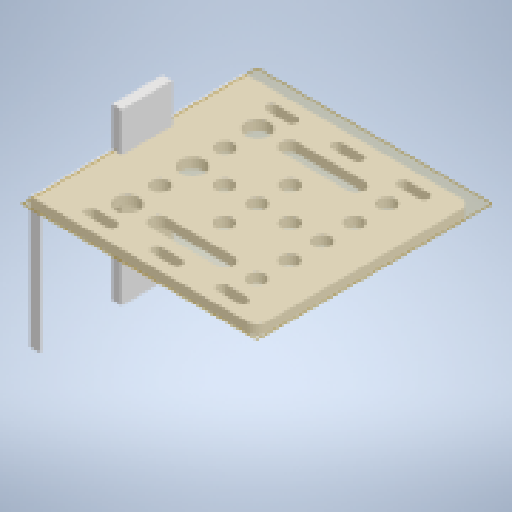
# Autodesk Inventor part: деталь основа каретки
Saved by Autodesk Inventor 2024.2 (Build 282272000, 272)
## iProperties
Created: 2026-01-31
Part Number: деталь основа каретки
Material: Типовые
Document SubType Name: Modeling
Designer: katya_notebook
Density: 1 g/cm^3
Appearance: По умолчанию
Author: katya_notebook
Autodesk Inventor part; units mm, degrees
ref_plane "YZ Plane" through (0, 0, 0) normal (1, 0, 0) x (0, 1, 0)
ref_plane "XZ Plane" through (0, 0, 0) normal (0, 1, 0) x (-1, 0, 0)
ref_plane "XY Plane" through (0, 0, 0) normal (0, 0, 1) x (1, 0, 0)
ref_plane "РабПлоскость1" through (-66.9457, 3.4254, 42.3112) normal (0, 1, 0) x (-1, 0, 0)
sketch "Эскиз1" plane through (-66.9457, 3.4254, 42.3112) normal (0, 1, 0) x (-1, 0, 0)
  arc A0 (3, 0) -> (0, 3) centre (0, 0) ccw projected
  line L0 (0, 3) -> (-59.5, 3) projected
  arc A1 (-59.5, 3) -> (-62.5, 0) centre (-59.5, 0) ccw projected
  line L1 (-62.5, 0) -> (-62.5, -59.5) projected
  arc A2 (-62.5, -59.5) -> (-59.5, -62.5) centre (-59.5, -59.5) ccw projected
  line L2 (-59.5, -62.5) -> (0, -62.5) projected
  arc A3 (0, -62.5) -> (3, -59.5) centre (0, -59.5) ccw projected
  line L3 (3, -59.5) -> (3, 0) projected
  circle A4 centre (-29.75, -29.75) radius 2.55 projected
  circle A5 centre (-39.75, -29.75) radius 2.55 projected
  circle A6 centre (-9.9, -49.75) radius 3.6 projected
  circle A7 centre (-9.9, -9.75) radius 3.6 projected
  circle A8 centre (-49.6, -49.75) radius 2.55 projected
  circle A9 centre (-49.6, -9.75) radius 2.55 projected
  circle A10 centre (-49.6, -39.75) radius 2.55 projected
  circle A11 centre (-9.9, -19.75) radius 2.55 projected
  arc A12 (-33, -55.95) -> (-33, -58.95) centre (-33, -57.45) ccw projected
  line L4 (-26.5, -55.95) -> (-33, -55.95) projected
  arc A13 (-26.5, -58.95) -> (-26.5, -55.95) centre (-26.5, -57.45) ccw projected
  line L5 (-33, -58.95) -> (-26.5, -58.95) projected
  arc A14 (-46.65, -58.95) -> (-46.65, -55.95) centre (-46.65, -57.45) ccw projected
  line L6 (-53.15, -58.95) -> (-46.65, -58.95) projected
  arc A15 (-53.15, -55.95) -> (-53.15, -58.95) centre (-53.15, -57.45) ccw projected
  line L7 (-46.65, -55.95) -> (-53.15, -55.95) projected
  arc A16 (-12.85, -0.55) -> (-12.85, -3.55) centre (-12.85, -2.05) ccw projected
  line L8 (-6.35, -0.55) -> (-12.85, -0.55) projected
  arc A17 (-6.35, -3.55) -> (-6.35, -0.55) centre (-6.35, -2.05) ccw projected
  line L9 (-12.85, -3.55) -> (-6.35, -3.55) projected
  arc A18 (-46.65, -3.55) -> (-46.65, -0.55) centre (-46.65, -2.05) ccw projected
  line L10 (-53.15, -3.55) -> (-46.65, -3.55) projected
  arc A19 (-53.15, -0.55) -> (-53.15, -3.55) centre (-53.15, -2.05) ccw projected
  line L11 (-46.65, -0.55) -> (-53.15, -0.55) projected
  arc A20 (-33, -0.55) -> (-33, -3.55) centre (-33, -2.05) ccw projected
  line L12 (-26.5, -0.55) -> (-33, -0.55) projected
  arc A21 (-26.5, -3.55) -> (-26.5, -0.55) centre (-26.5, -2.05) ccw projected
  line L13 (-33, -3.55) -> (-26.5, -3.55) projected
  arc A22 (-40.07, -7.25) -> (-40.07, -12.25) centre (-40.07, -9.75) ccw projected
  line L14 (-19.43, -7.25) -> (-40.07, -7.25) projected
  arc A23 (-19.43, -12.25) -> (-19.43, -7.25) centre (-19.43, -9.75) ccw projected
  line L15 (-40.07, -12.25) -> (-19.43, -12.25) projected
  arc A24 (-12.85, -55.95) -> (-12.85, -58.95) centre (-12.85, -57.45) ccw projected
  line L16 (-6.35, -55.95) -> (-12.85, -55.95) projected
  arc A25 (-6.35, -58.95) -> (-6.35, -55.95) centre (-6.35, -57.45) ccw projected
  line L17 (-12.85, -58.95) -> (-6.35, -58.95) projected
  arc A26 (-40.07, -47.25) -> (-40.07, -52.25) centre (-40.07, -49.75) ccw projected
  line L18 (-19.43, -47.25) -> (-40.07, -47.25) projected
  arc A27 (-19.43, -52.25) -> (-19.43, -47.25) centre (-19.43, -49.75) ccw projected
  line L19 (-40.07, -52.25) -> (-19.43, -52.25) projected
  circle A28 centre (-49.6, -19.75) radius 2.55 projected
  circle A29 centre (-29.75, -19.75) radius 2.55 projected
  circle A30 centre (-49.6, -29.75) radius 2.55 projected
  circle A31 centre (-9.9, -39.75) radius 2.55 projected
  circle A32 centre (-9.9, -29.75) radius 3.6 projected
  circle A33 centre (-19.75, -29.75) radius 2.55 projected
  circle A34 centre (-29.75, -39.75) radius 2.55 projected
  line L20 (3, -59.5) -> (3, -62.5)
  line L21 (3, -62.5) -> (0, -62.5)
  line L22 (0, 3) -> (3, 3)
  line L23 (3, 3) -> (3, 0)
  point P0 (-66.9457, -42.3112)
  constraints: 8 end point, 2 perpendicular, 1 horizontal, 1 tangent, 1 vertical
extrude "Выдавливание1" add sketch "Эскиз1" against normal blind 3
sketch "Эскиз3" plane through (-66.9457, 3.4254, 42.3112) normal (0, 1, 0) x (1, 0, 0)
  line L0 (59.5, -3) -> (-3, -3) projected
  line L1 (-3, -3) -> (-7, -3)
  line L2 (-7, -3) -> (-7, 62.5)
  line L3 (-7, 62.5) -> (-3, 62.5)
  line L4 (-3, 62.5) -> (-3, -3)
  point P0 (66.9457, 42.3112)
  dimension "d5" = 4
  constraints: 8 end point, 2 parallel, 1 horizontal, 1 perpendicular
  measures "d5" distance of L2.end L3.end
extrude "Выдавливание3" add sketch "Эскиз3" against normal blind 3
sketch "Эскиз4" plane through (-66.9457, 3.4254, 42.3112) normal (0, 1, 0) x (1, 0, 0)
  line L0 (-7, 62.5) -> (59.5, 62.5) projected
  line L1 (59.5, -3) -> (-7, -3) projected
  line L2 (-7, 62.5) -> (-4, 62.5)
  line L3 (-4, 62.5) -> (-4, -3)
  line L4 (-4, -3) -> (-7, -3)
  line L5 (-7, -3) -> (-7, 62.5)
  point P0 (66.9457, 42.3112)
  point P1 (-4, 62.5)
  dimension "d8" = 3
  constraints: 8 end point, 2 parallel, 1 horizontal, 1 perpendicular, 1 point on line
  measures "d8" distance between parallel lines of L3 L5
extrude "Выдавливание4" add sketch "Эскиз4" along normal blind 12 and the other way blind 40
sketch "Эскиз9" plane through (-66.9457, 15.4254, 42.3112) normal (0, 1, 0) x (1, 0, 0)
  line L0 (-7, 62.5) -> (-4, 62.5) projected
  line L1 (-4, 62.5) -> (-7, 62.5)
  line L2 (-7, 62.5) -> (-7, 37.5)
  line L3 (-7, 37.5) -> (-4, 37.5)
  line L4 (-4, 37.5) -> (-4, 62.5)
  line L5 (-4, -3) -> (-7, -3) projected
  line L6 (-7, 22) -> (-4, 22)
  line L7 (-4, 22) -> (-4, -3)
  line L8 (-4, -3) -> (-7, -3)
  line L9 (-7, -3) -> (-7, 22)
  point P0 (66.9457, 42.3112)
  point P1 (-7, 62.5)
  dimension "d24" = 25
  dimension "d25" = 25
  constraints: 16 end point, 4 parallel, 2 horizontal, 2 perpendicular, 1 point on line
  measures "d24" distance of L3.end L0.end
  measures "d25" distance of L6.end L5.start
extrude "Выдавливание8" cut sketch "Эскиз9" against normal blind 12
sketch "Эскиз10" plane through (-66.9457, -36.5746, 42.3112) normal (0, -1, 0) x (1, 0, 0)
  line L0 (-7, 3) -> (-7, -62.5) projected
  line L1 (-4, -37.5) -> (-7, -37.5) projected
  line L2 (-7, -62.5) -> (-4, -62.5)
  line L3 (-4, -62.5) -> (-4, -37.5)
  line L4 (-4, -37.5) -> (-7, -37.5)
  line L5 (-7, -37.5) -> (-7, -62.5)
  line L6 (-7, -22) -> (-4, -22) projected
  line L7 (-7, 2.6439) -> (-4, 2.6439)
  line L8 (-4, 2.6439) -> (-4, -22)
  line L9 (-4, -22) -> (-7, -22)
  line L10 (-7, -22) -> (-7, 2.6439)
  point P0 (66.9457, -42.3112)
  point P1 (-7, 2.6439)
  constraints: 16 end point, 4 parallel, 2 horizontal, 2 perpendicular, 1 point on line
extrude "Выдавливание9" cut sketch "Эскиз10" against normal blind 37
fillet "Сопряжение4" radius 4 4 edges at (-72.4457, 3.4254, 4.8112) (-72.4457, 0.4254, 4.8112) (-72.4457, 3.4254, 20.3112) (-72.4457, 0.4254, 20.3112)
fillet "Сопряжение5" radius 6 6 edges at (-70.9457, 3.4254, 2.8112) (-70.9457, 3.4254, 12.5612) (-70.9457, 3.4254, 22.3112) (-70.9457, 0.4254, 22.3112) (-70.9457, 0.4254, 12.5612) (-70.9457, 0.4254, 2.8112)
sketch "Эскиз11" plane through (-73.9457, -36.5746, 45.3112) normal (-1, 0, 0) x (0, 0, 1)
  circle A0 centre (-32.75, 47.5) radius 1.2 projected
  circle A1 centre (-32.75, 32.5) radius 1.2 projected
  circle A2 centre (-32.75, 17.5) radius 1.2 projected
  circle A3 centre (-32.75, 2.5) radius 1.2 projected
  point P0 (-45.3112, 36.5746)
extrude "Выдавливание10" cut sketch "Эскиз11" against normal blind 37
